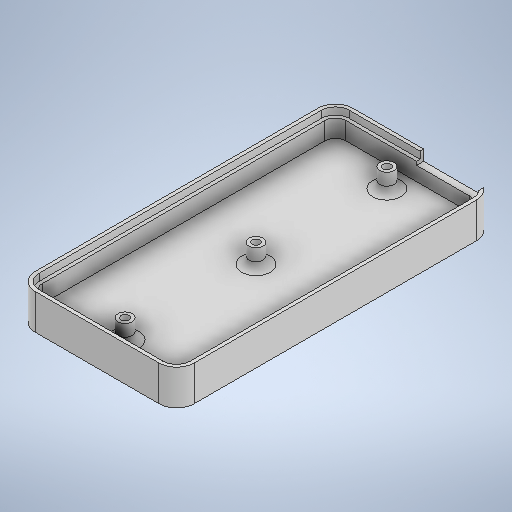
# Autodesk Inventor part: Pieza_baja
Saved by Autodesk Inventor 2025.1 (Build 291241000, 241)
## iProperties
Created: 2024-08-25
Part Number: Pieza_baja
Material: Genérico
Document SubType Name: Modeling
Designer: User
Density: 1 g/cm^3
Appearance: Valor por defecto
Author: User
Autodesk Inventor part; units mm, degrees
ref_plane "YZ Plane" through (0, 0, 0) normal (1, 0, 0) x (0, 1, 0)
ref_plane "XZ Plane" through (0, 0, 0) normal (0, 1, 0) x (-1, 0, 0)
ref_plane "XY Plane" through (0, 0, 0) normal (0, 0, 1) x (1, 0, 0)
sketch "Boceto1" plane through (0, 0, 0) normal (0, 1, 0) x (-1, 0, 0)
  line L0 (17.5, 45) -> (-17.5, 45)
  line L1 (-22.5, 40) -> (-22.5, -40)
  line L2 (-17.5, -45) -> (17.5, -45)
  line L3 (22.5, -40) -> (22.5, 40)
  line L4 (22.5, 45) -> (-22.5, -45) construction
  line L5 (-22.5, 45) -> (22.5, -45) construction
  arc A0 (22.5, 40) -> (17.5, 45) centre (17.5, 40) ccw
  arc A1 (-17.5, 45) -> (-22.5, 40) centre (-17.5, 40) ccw
  arc A2 (-22.5, -40) -> (-17.5, -45) centre (-17.5, -40) ccw
  arc A3 (17.5, -45) -> (22.5, -40) centre (17.5, -40) ccw
  point P0 (0, 0)
  dimension "d0" = 45
  dimension "d1" = 90
  dimension "d2" = 5
  constraints: 12 end point, 8 point on circle, 8 point on line, 8 tangent, 4 centre point, 3 equal radius, 2 midpoint, 2 parallel, 1 horizontal, 1 perpendicular
  measures "d0" distance of L5.end L4.end
  measures "d1" distance of L4.end L5.start
  measures "d2" radius of A0
extrude "Extrusión1" add sketch "Boceto1" along normal blind 10
sketch "Boceto2" plane through (0, 10, 0) normal (0, 1, 0) x (1, 0, 0)
  arc A0 (17.5, -45) -> (22.5, -40) centre (17.5, -40) ccw projected
  line L0 (22.5, -40) -> (22.5, 40) projected
  arc A1 (22.5, 40) -> (17.5, 45) centre (17.5, 40) ccw projected
  line L1 (17.5, 45) -> (-17.5, 45) projected
  arc A2 (-17.5, 45) -> (-22.5, 40) centre (-17.5, 40) ccw projected
  line L2 (-22.5, 40) -> (-22.5, -40) projected
  arc A3 (-22.5, -40) -> (-17.5, -45) centre (-17.5, -40) ccw projected
  line L3 (-17.5, -45) -> (17.5, -45) projected
  arc A4 (-21.5, -40) -> (-17.5, -44) centre (-17.5, -40) ccw
  line L4 (-21.5, -40) -> (-21.5, 40)
  arc A5 (-17.5, 44) -> (-21.5, 40) centre (-17.5, 40) ccw
  line L5 (-17.5, 44) -> (17.5, 44)
  arc A6 (21.5, 40) -> (17.5, 44) centre (17.5, 40) ccw
  line L6 (21.5, 40) -> (21.5, -40)
  arc A7 (17.5, -44) -> (21.5, -40) centre (17.5, -40) ccw
  line L7 (17.5, -44) -> (-17.5, -44)
  line L8 (-20.5, 40) -> (-20.5, -40)
  arc A8 (-20.5, -40) -> (-17.5, -43) centre (-17.5, -40) ccw
  line L9 (-17.5, -43) -> (17.5, -43)
  arc A9 (17.5, -43) -> (20.5, -40) centre (17.5, -40) ccw
  line L10 (20.5, -40) -> (20.5, 40)
  arc A10 (20.5, 40) -> (17.5, 43) centre (17.5, 40) ccw
  line L11 (17.5, 43) -> (-17.5, 43)
  arc A11 (-17.5, 43) -> (-20.5, 40) centre (-17.5, 40) ccw
  point P0 (0, 0)
  dimension "d5" = 1
  dimension "d6" = 1
  constraints: 16 end point, 16 point on circle, 8 centre point, 14 other
  measures "d5" radial gap between concentric circles of A3 A4
  measures "d6" distance between parallel lines of L4 L8
extrude "Extrusión2" cut sketch "Boceto2" against normal blind 2 contours L4 A5 L5 A6 L6 A7 L7 A4
sketch "Boceto3" plane through (0, 10, 0) normal (0, 1, 0) x (1, 0, 0)
  line L0 (17.5, 43) -> (-17.5, 43) projected
  arc A0 (-17.5, 43) -> (-20.5, 40) centre (-17.5, 40) ccw projected
  line L1 (-20.5, 40) -> (-20.5, -40) projected
  arc A1 (-20.5, -40) -> (-17.5, -43) centre (-17.5, -40) ccw projected
  line L2 (-17.5, -43) -> (17.5, -43) projected
  arc A2 (17.5, -43) -> (20.5, -40) centre (17.5, -40) ccw projected
  line L3 (20.5, -40) -> (20.5, 40) projected
  arc A3 (20.5, 40) -> (17.5, 43) centre (17.5, 40) ccw projected
  point P0 (0, 0)
extrude "Extrusión3" cut sketch "Boceto3" against normal blind 7
sketch "Boceto4" plane through (0, 3, 0) normal (0, 1, 0) x (1, 0, 0)
  circle A0 centre (0, 0) radius 2
  circle A1 centre (0, 0) radius 1.1
  dimension "d11" = 4
  dimension "d12" = 2.2
  constraints: 2 centre point, 2 coincident
  measures "d11" diameter of A0
  measures "d12" diameter of A1
extrude "Extrusión4" add sketch "Boceto4" along normal blind 5.4
fillet "Empalme1" radius 2 1 edges at (-2, 3, 0)
sketch "Boceto5" plane through (0, 3, 0) normal (0, 1, 0) x (1, 0, 0)
  line L0 (17.5, -43) -> (-17.5, -43) construction
  line L1 (0, -43) -> (0, -37.1) construction
  line L2 (-17.5, 43) -> (17.5, 43) construction
  line L3 (0, 43) -> (0, 37.1) construction
  circle A0 centre (0, -37.1) radius 2
  circle A1 centre (0, -37.1) radius 1.1
  circle A2 centre (0, 37.1) radius 2
  circle A3 centre (0, 37.1) radius 1.1
  point P0 (0, 0)
  dimension "d16" = 5.9
  dimension "d17" = 5.9
  dimension "d18" = 4
  dimension "d19" = 2.2
  dimension "d20" = 4
  dimension "d21" = 2.2
  constraints: 4 centre point, 4 coincident, 4 end point, 2 midpoint, 2 vertical
  measures "d16" distance of L1.start L1.end
  measures "d17" distance of L3.start L3.end
  measures "d18" diameter of A0
  measures "d19" diameter of A1
  measures "d20" diameter of A2
  measures "d21" diameter of A3
extrude "Extrusión5" add sketch "Boceto5" along normal blind 5.4
fillet "Empalme2" radius 2 2 edges at (-2, 3, 37.1) (-2, 3, -37.1)
sketch "Sketch10" plane through (17.5, 0, -45) normal (0, 0, -1) x (-1, 0, 0)
  line L0 (-3.0024, 10) -> (14.9976, 10)
  line L1 (14.9976, 10) -> (14.9976, 7)
  line L2 (14.9976, 7) -> (-3.0024, 7)
  line L3 (-3.0024, 7) -> (-3.0024, 10)
  point P0 (17.5, 0)
  dimension "d37" = 18
  dimension "d38" = 3
  constraints: 8 end point, 2 parallel, 1 horizontal, 1 perpendicular
  measures "d37" distance of L1.end L2.end
  measures "d38" distance of L0.end L1.end
extrude "Extrusion10" cut sketch "Sketch10" against normal blind 5
